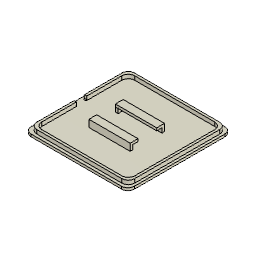
lid (Autodesk Fusion 360 design; units mm, degrees)
part number: 2025-11-17-17-24-12-968
Autodesk Fusion 360 part; units mm, degrees
sketch "Sketch1" plane through (0, 0, 0) normal (0, 0, 1) x (1, 0, 0)
box "BoxPrimitive1" add length 80 width 80 height 2 placed x (0, 1, 0) y (-1, 0, 0) z (0, 0, 1) at (80, 0, 0)
sketch "Sketch3" plane through (0, 0, 2) normal (0, 0, 1) x (-1, 0, 0)
  line L0 (-80, -80) -> (0, -80)
  line L1 (0, -80) -> (0, 0)
  line L2 (0, 0) -> (-80, 0)
  line L3 (-80, 0) -> (-80, -80)
  line L4 (-0.1, -80.1) -> (-80.1, -80.1)
  line L5 (-80.1, -80.1) -> (-80.1, -0.1)
  line L6 (-80.1, -0.1) -> (-0.1, -0.1)
  line L7 (-0.1, -0.1) -> (-0.1, -80.1)
  line L8 (-0.1, -80.1) -> (-80.1, -0.1) construction
  line L9 (-80.1, -80.1) -> (-0.1, -0.1) construction
  line L10 (-2.2, -78) -> (-78, -78)
  line L11 (-78, -78) -> (-78, -2.2)
  line L12 (-78, -2.2) -> (-2.2, -2.2)
  line L13 (-2.2, -2.2) -> (-2.2, -78)
  line L14 (-2.2, -78) -> (-78, -2.2) construction
  line L15 (-78, -78) -> (-2.2, -2.2) construction
  line L16 (-4.1, -76.1) -> (-76.1, -76.1)
  line L17 (-76.1, -76.1) -> (-76.1, -4.1)
  line L18 (-76.1, -4.1) -> (-4.1, -4.1)
  line L19 (-4.1, -4.1) -> (-4.1, -76.1)
  line L20 (-4.1, -76.1) -> (-76.1, -4.1) construction
  line L21 (-76.1, -76.1) -> (-4.1, -4.1) construction
  point P0 (-40.1, -40.1)
  point P1 (-40.1, -40.1)
  point P2 (-40.1, -40.1)
  dimension "d8" = 80
  dimension "d9" = 80
  dimension "d10" = 75.8
  dimension "d11" = 75.8
  dimension "d12" = 72
  dimension "d13" = 72
  constraint horizontal L4
  constraint perpendicular L4 L5
  constraint parallel L4 L6
  constraint parallel L5 L7
  constraint coincident L8 P2
  constraint coincident L9 P2
  constraint horizontal L10
  constraint perpendicular L10 L11
  constraint parallel L10 L12
  constraint parallel L11 L13
  constraint coincident L14 P2
  constraint coincident L15 P2
  constraint coincident P2 P1
  constraint horizontal L16
  constraint perpendicular L16 L17
  constraint parallel L16 L18
  constraint parallel L17 L19
  constraint coincident L20 P2
  constraint coincident L21 P2
  measures "d8" distance of L5.end L6.end
  measures "d9" distance of L4.end L5.end
  measures "d10" distance of L11.end L12.end
  measures "d11" distance of L10.end L11.end
  measures "d12" distance of L17.end L18.end
  measures "d13" distance of L16.end L17.end
extrude "Extrude1" add sketch "Sketch3" along normal blind 3 contours L10 L11 L12 L13
fillet "Fillet1" radius 5 12 edges at (80, 0, 1) (80, 80, 1) (78, 78, 3.5) (78, 2.2, 3.5) (2.2, 78, 3.5) (0, 80, 1) (2.2, 2.2, 3.5) (0, 0, 1) (76.1, 4.1, 3.5) (76.1, 76.1, 3.5) (4.1, 76.1, 3.5) (4.1, 4.1, 3.5)
sketch "Sketch4" plane through (0, 0, 0) normal (1, 0, 0) x (0, 1, 0)
  line L0 (80, 0) -> (0, 0)
  line L1 (44, 7) -> (36, 7)
  line L2 (44, 12) -> (36, 12)
  line L3 (36, 12) -> (36, 2)
  line L4 (36, 2) -> (44, 2)
  line L5 (44, 2) -> (44, 12)
  line L6 (44, 12) -> (36, 2) construction
  line L7 (36, 12) -> (44, 2) construction
  point P0 (40, 7)
  point P1 (40, 7)
  dimension "d24" = 8
  dimension "d25" = 10
  constraint coincident L0.end origin
  constraint horizontal L0
  constraint horizontal L2
  constraint perpendicular L2 L3
  constraint parallel L2 L4
  constraint parallel L3 L5
  constraint coincident L6 P1
  constraint coincident L7 P1
  constraint coincident P1 P0
  measures "d24" distance of L3.end L4.end
  measures "d25" distance of L2.end L3.end
extrude "Extrude2" cut sketch "Sketch4" along normal blind 5 contours L1 L3 L4 L5
fillet "Fillet2" radius 0.5 2 edges at (3.15, 44, 2) (3.15, 36, 2)
sketch "Sketch5" plane through (0, 0, 2) normal (0, 0, 1) x (-1, 0, 0)
  line L0 (-55, -51.25) -> (-25, -51.25)
  line L1 (-25, -51.25) -> (-25, -28.75)
  line L2 (-25, -28.75) -> (-55, -28.75)
  line L3 (-55, -28.75) -> (-55, -51.25)
  line L4 (-55, -51.25) -> (-25, -28.75) construction
  line L5 (-25, -51.25) -> (-55, -28.75) construction
  line L6 (-55, -40) -> (-25, -40) construction
  line L7 (-40, -51.25) -> (-40, -28.75) construction
  line L8 (-40, -51.25) -> (-40, -49.25) construction
  line L9 (-40, -49.25) -> (-55, -49.25)
  line L10 (-40, -49.25) -> (-25, -49.25)
  point P0 (-40, -40)
  dimension "d28" = 30
  dimension "d29" = 22.5
  dimension "d30" = 2
  constraint horizontal L0
  constraint perpendicular L0 L1
  constraint parallel L0 L2
  constraint parallel L1 L3
  constraint coincident L4 P0
  constraint coincident L5 P0
  constraint midpoint L3 L6.start
  constraint midpoint L1 L6.end
  constraint midpoint L0 L7.start
  constraint midpoint L2 L7.end
  constraint perpendicular L0 L8
  constraint coincident L3 L9.end
  constraint perpendicular L3 L9
  constraint coincident L1 L10.end
  constraint perpendicular L1 L10
  measures "d28" distance of L1.end L2.end
  measures "d29" distance of L0.end L1.end
  measures "d30" distance of L7.start L8.end
ref_plane "WorkPlane1" through (25, 40, 1) normal (-1, 0, 0) x (0, 0, 1)
ref_plane "WorkPlane2" through (55, 40, 1) normal (-1, 0, 0) x (0, 0, 1)
sketch "Sketch6" plane through (25, 0, 0) normal (-1, 0, 0) x (0, -1, 0)
  line L0 (-40, 2) -> (-53.25, 2)
  line L1 (-40, 2) -> (-49.25, 2)
  line L2 (-53.25, 2) -> (-53.25, 7.5)
  line L3 (-53.25, 7.5) -> (-47.25, 7.5)
  line L4 (-53.25, 2) -> (-51.25, 2)
  line L5 (-51.25, 2) -> (-51.25, 5.5)
  line L6 (-51.25, 5.5) -> (-47.25, 5.5)
  line L7 (-47.25, 7.5) -> (-47.25, 5.5)
  line L8 (-47.25, 5.5) -> (-47.25, 2)
  point P0 (-40, 2)
  point P1 (-49.25, 2)
  dimension "d33" = 13.25
  dimension "d34" = 5.5
  dimension "d35" = 6
  dimension "d37" = 2
  dimension "d47" = 3.5
  dimension "d48" = 4
  constraint coincident P0 L0.start
  constraint coincident P1 L1.end
  constraint perpendicular L0 L2
  constraint perpendicular L2 L3
  constraint perpendicular L2 L4
  constraint perpendicular L4 L5
  constraint perpendicular L5 L6
  constraint coincident L0 L8.end
  constraint perpendicular L0 L8
  measures "d33" distance of P0 L0.end
  measures "d34" distance of L0.end L2.end
  measures "d35" distance of L2.end L3.end
  measures "d37" distance of L0.end L4.end
  measures "d47" distance of L4.end L5.end
  measures "d48" distance of L5.end L6.end
extrude "Extrude3" add sketch "Sketch6" along normal blind -30 and the other way blind -2 contours L0 L2 L3 L4 L5 L6 L7
extrude "Extrude4" add sketch "Sketch6" along normal blind 2 contours L0 L1 L5 L6 L8
ref_plane "WorkPlane3" through (40, 40, 1) normal (0, 1, 0) x (0, 0, -1)
mirror "Mirror1" about plane through (40, 40, 1) normal (0, 1, 0) of "Extrude3", "Extrude4"
